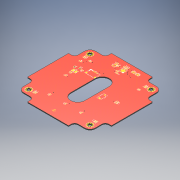
# Autodesk Inventor part: -ZPanel_PCB
Saved by Autodesk Inventor 2018 (Build 220112000, 112)
## iProperties
Created: 2018-11-03
Part Number: -ZPanel_PCB
Material: Epoxy Resin
Document SubType Name: Modeling
Designer: Bradley
Density: 1.14 g/cm^3
Appearance: Smooth - Dark Gray
Mass: 5.79181 g
Surface Area: 172.339 cm^2
Volume: 5.08053 cm^3
Author: Bradley
Autodesk Inventor part; units mm, degrees
ref_plane "YZ Plane" through (0, 0, 0) normal (1, 0, 0) x (0, 1, 0)
ref_plane "XZ Plane" through (0, 0, 0) normal (0, 1, 0) x (-1, 0, 0)
ref_plane "XY Plane" through (0, 0, 0) normal (0, 0, 1) x (1, 0, 0)
sketch "Sketch1" plane through (0, 0, 0) normal (0, 0, 1) x (1, 0, 0)
  line L0 (-48, -48) -> (48, -48)
  line L1 (48, -48) -> (48, 48)
  line L2 (48, 48) -> (-48, 48)
  line L3 (-48, 48) -> (-48, -48)
  line L4 (-48, -48) -> (48, 48) construction
  line L5 (48, -48) -> (-48, 48) construction
  circle A0 centre (0, 0) radius 40 construction
  circle A1 centre (0, 0) radius 8
  line L6 (-45, -32.5) -> (45, -32.5) construction
  line L7 (45, -32.5) -> (45, 32.5) construction
  line L8 (45, 32.5) -> (-45, 32.5) construction
  line L9 (-45, 32.5) -> (-45, -32.5) construction
  line L10 (-45, -32.5) -> (45, 32.5) construction
  line L11 (45, -32.5) -> (-45, 32.5) construction
  line L12 (-28, -46.5) -> (28, -46.5) construction
  line L13 (28, -46.5) -> (28, 46.5) construction
  line L14 (28, 46.5) -> (-28, 46.5) construction
  line L15 (-28, 46.5) -> (-28, -46.5) construction
  line L16 (-28, -46.5) -> (28, 46.5) construction
  line L17 (28, -46.5) -> (-28, 46.5) construction
  circle A2 centre (-45, 32.5) radius 4 construction
  circle A3 centre (-28, 46.5) radius 4 construction
  line L18 (-35, -35) -> (35, -35) construction
  line L19 (35, -35) -> (35, 35) construction
  line L20 (35, 35) -> (-35, 35) construction
  line L21 (-35, 35) -> (-35, -35) construction
  line L22 (-35, -35) -> (35, 35) construction
  line L23 (35, -35) -> (-35, 35) construction
  circle A4 centre (-35, 35) radius 3 construction
  line L24 (-23.5, 48) -> (-23.5, 45)
  arc A5 (-27.5, 41) -> (-23.5, 45) centre (-27.5, 45) ccw
  line L25 (-27.5, 41) -> (-35, 41)
  arc A6 (-35, 41) -> (-41, 35) centre (-35, 35) ccw
  line L26 (-41, 35) -> (-41, 27.5)
  arc A7 (-45, 23.5) -> (-41, 27.5) centre (-45, 27.5) ccw
  line L27 (-45, 23.5) -> (-48, 23.5)
  line L28 (48, 23.5) -> (45, 23.5)
  arc A8 (41, 27.5) -> (45, 23.5) centre (45, 27.5) ccw
  line L29 (41, 27.5) -> (41, 35)
  arc A9 (41, 35) -> (35, 41) centre (35, 35) ccw
  line L30 (35, 41) -> (27.5, 41)
  arc A10 (23.5, 45) -> (27.5, 41) centre (27.5, 45) ccw
  line L31 (23.5, 45) -> (23.5, 48)
  line L32 (48, -23.5) -> (45, -23.5)
  arc A11 (45, -23.5) -> (41, -27.5) centre (45, -27.5) ccw
  line L33 (41, -27.5) -> (41, -35)
  arc A12 (35, -41) -> (41, -35) centre (35, -35) ccw
  line L34 (35, -41) -> (27.5, -41)
  arc A13 (27.5, -41) -> (23.5, -45) centre (27.5, -45) ccw
  line L35 (23.5, -45) -> (23.5, -48)
  line L36 (-23.5, -48) -> (-23.5, -45)
  arc A14 (-23.5, -45) -> (-27.5, -41) centre (-27.5, -45) ccw
  line L37 (-27.5, -41) -> (-35, -41)
  arc A15 (-41, -35) -> (-35, -41) centre (-35, -35) ccw
  line L38 (-41, -35) -> (-41, -27.5)
  arc A16 (-41, -27.5) -> (-45, -23.5) centre (-45, -27.5) ccw
  line L39 (-45, -23.5) -> (-48, -23.5)
  line L40 (0, 14) -> (0, -14) construction
  line L41 (8, 14) -> (8, -14)
  line L42 (-8, -14) -> (-8, 14)
  arc A17 (8, 14) -> (-8, 14) centre (0, 14) ccw
  arc A18 (-8, -14) -> (8, -14) centre (0, -14) ccw
  dimension "d0" = 96
  dimension "d1" = 96
  dimension "d3" = 80
  dimension "d7" = 16
  dimension "d48" = 90
  dimension "d49" = 65
  dimension "d50" = 56
  dimension "d51" = 93
  dimension "d52" = 8
  dimension "d53" = 70
  dimension "d54" = 6
  dimension "d55" = 23.5
  dimension "d56" = 23.5
  dimension "d57" = 4
  dimension "d58" = 41
  dimension "d59" = 28
  constraints: 86 end point, 28 point on circle, 28 tangent, 19 centre point, 17 perpendicular, 11 equal radius, 11 point on line, 9 midpoint, 8 parallel, 7 collinear, 6 horizontal, 5 coincident, 4 equal length, 3 vertical, 1 concentric, 3 other
  measures "d0" distance of L2.end L1.end
  measures "d1" distance of L1.end L0.end
  measures "d3" diameter of A0
  measures "d7" diameter of A1
  measures "d48" distance of L8.end L7.end
  measures "d49" distance of L7.end L6.end
  measures "d50" distance of L14.end L14.start
  measures "d51" distance of L14.start L12.end
  measures "d52" diameter of A2
  measures "d53" distance of L20.end L19.end
  measures "d54" diameter of A4
  measures "d55" distance from line of point (0, 0) L24
  measures "d56" distance from line of point (0, 0) L27
  measures "d57" radius of A5
  measures "d58" distance from line of point (0, 0) L26
  measures "d59" distance of L41.start L41.end
extrude "Extrusion1" add sketch "Sketch1" along normal mid plane 1 contours L36 A14 L37 A15 L38 A16 L39 L3 L27 A7 L26 A6 L25 A5 L24 L2 L31 A10 L30 A9 L29 A8 L28 L1 L32 A11 L33 A12 L34 A13 L35 L0
fillet "Fillet1" radius 0.5 8 edges at (-23.5, -48, 0) (-48, -23.5, 0) (-48, 23.5, 0) (-23.5, 48, 0) (23.5, 48, 0) (48, 23.5, 0) (48, -23.5, 0) (23.5, -48, 0)
sketch "Sketch4" plane through (0, 0, 0.5) normal (0, 0, 1) x (1, 0, 0)
  line L0 (-35, -35) -> (35, -35) construction
  line L1 (35, -35) -> (35, 35) construction
  line L2 (35, 35) -> (-35, 35) construction
  line L3 (-35, 35) -> (-35, -35) construction
  line L4 (-35, -35) -> (35, 35) construction
  line L5 (35, -35) -> (-35, 35) construction
  point P0 (0, 0)
  dimension "d35" = 70
  constraints: 12 end point, 4 coincident, 2 midpoint, 2 parallel, 2 perpendicular, 1 horizontal
  measures "d35" distance of L2.end L1.end
hole "Hole3" at (-35, 35, 0.5) at (35, 35, 0.5) at (35, -35, 0.5) at (-35, -35, 0.5) direction (0, 0, -1) diameter 3.4 end through all clearance for "Flat Head Machine Screw" size "M3" standard "Ansi Metric M Profile"
sketch "Sketch13" plane through (0, 0, 0.5) normal (0, 0, 1) x (1, 0, 0)
  line L0 (-48, 48) -> (48, 48) construction
  line L1 (48, 48) -> (48, -48) construction
  line L2 (48, -48) -> (-48, -48) construction
  line L3 (-48, -48) -> (-48, 48) construction
  line L4 (23, 48) -> (-23, 48) projected
  line L5 (-23, -48) -> (23, -48) projected
  point P0 (0, 0)
  point P1 (0, 48)
  constraints: 2 collinear, 2 midpoint, 2 other
decal "Decal3"
sketch "Sketch8" plane through (0, 0, -0.5) normal (0, 0, -1) x (-1, 0, 0)
  line L0 (-48, 48) -> (48, 48) construction
  line L1 (48, 48) -> (48, -48) construction
  line L2 (48, -48) -> (-48, -48) construction
  line L3 (-48, -48) -> (-48, 48) construction
  line L4 (23, 48) -> (-23, 48) projected
  line L5 (-23, -48) -> (23, -48) projected
  point P0 (0, 0)
  point P1 (0, 48)
  constraints: 2 collinear, 2 midpoint, 2 other
decal "Decal2"
sketch "Sketch9" plane through (0, 0, 0.5) normal (0, 0, 1) x (1, 0, 0)
  point P0 (0, 0)
  point P1 (-26.75, 15.31)
  point P2 (-31.25, 13.5)
  constraints: 2 other
hole "Hole4" at (-26.75, 15.31, 0.5) at (-31.25, 13.5, 0.5) direction (0, 0, -1) diameter 0.7 end through all
sketch "Sketch10" plane through (0, 0, 0.5) normal (0, 0, 1) x (1, 0, 0)
  point P0 (0, 0)
  point P1 (35.711, -32.813)
  point P2 (34.289, -32.813)
  point P3 (33.139, -33.648)
  point P4 (32.7, -35)
  point P5 (34.289, -37.187)
  point P6 (35.711, -37.187)
  point P7 (36.861, -36.352)
  point P8 (37.3, 35)
  point P9 (-32.7, 35)
  point P10 (36.861, 36.352)
  point P11 (35.711, 37.187)
  point P12 (33.139, 36.352)
  point P13 (32.7, 35)
  point P14 (33.139, 33.648)
  point P15 (34.289, 32.813)
  point P16 (35.711, 32.813)
  point P17 (36.861, 33.648)
  point P18 (34.289, 37.187)
  point P19 (-32.7, -35)
  point P20 (-33.139, -33.648)
  point P21 (-34.289, -32.813)
  point P22 (-35.711, -32.813)
  point P23 (-36.861, -33.648)
  point P24 (-37.3, -35)
  point P25 (-36.861, -36.352)
  point P26 (-35.711, -37.187)
  point P27 (-34.289, -37.187)
  point P28 (-33.139, -36.352)
  point P29 (33.139, -36.352)
  point P30 (-33.139, 36.352)
  point P31 (-34.289, 37.187)
  point P32 (-35.711, 37.187)
  point P33 (-36.861, 36.352)
  point P34 (-37.3, 35)
  point P35 (-36.861, 33.648)
  point P36 (-35.711, 32.813)
  point P37 (-34.289, 32.813)
  point P38 (-33.139, 33.648)
  point P39 (37.3, -35)
  point P40 (36.861, -33.648)
  constraints: 41 other
hole "Hole5" at (35.711, -32.813, 0.5) at (34.289, -32.813, 0.5) at (33.139, -33.648, 0.5) at (32.7, -35, 0.5) at (34.289, -37.187, 0.5) at (35.711, -37.187, 0.5) at (36.861, -36.352, 0.5) at (37.3, 35, 0.5) at (-32.7, 35, 0.5) at (36.861, 36.352, 0.5) at (35.711, 37.187, 0.5) at (33.139, 36.352, 0.5) at (32.7, 35, 0.5) at (33.139, 33.648, 0.5) at (34.289, 32.813, 0.5) at (35.711, 32.813, 0.5) at (36.861, 33.648, 0.5) at (34.289, 37.187, 0.5) at (-32.7, -35, 0.5) at (-33.139, -33.648, 0.5) at (-34.289, -32.813, 0.5) at (-35.711, -32.813, 0.5) at (-36.861, -33.648, 0.5) at (-37.3, -35, 0.5) at (-36.861, -36.352, 0.5) at (-35.711, -37.187, 0.5) at (-34.289, -37.187, 0.5) at (-33.139, -36.352, 0.5) at (33.139, -36.352, 0.5) at (-33.139, 36.352, 0.5) at (-34.289, 37.187, 0.5) at (-35.711, 37.187, 0.5) at (-36.861, 36.352, 0.5) at (-37.3, 35, 0.5) at (-36.861, 33.648, 0.5) at (-35.711, 32.813, 0.5) at (-34.289, 32.813, 0.5) at (-33.139, 33.648, 0.5) at (37.3, -35, 0.5) at (36.861, -33.648, 0.5) direction (0, 0, -1) diameter 0.45 end through all
sketch "Sketch11" plane through (0, 0, 0.5) normal (0, 0, 1) x (1, 0, 0)
  point P0 (0, 0)
  point P1 (-11.75, 22.5)
  point P2 (-30.25, 22.5)
  point P3 (-4.025, 32.275)
  point P4 (-6.25, 34.75)
  point P5 (-29.5, 25.5)
  point P6 (-8, 23.5)
  point P7 (-6, 39.75)
  point P8 (5.25, 42.5)
  point P9 (2.5, 41.25)
  point P10 (-25, 28)
  point P11 (4.25, 39)
  point P12 (-25.75, 0)
  point P13 (4.75, 38)
  point P14 (-18, -23.5)
  point P15 (6, 37)
  point P16 (2, -25.25)
  point P17 (6.75, 36)
  point P18 (-11.75, 42.75)
  point P19 (25, 1.5)
  point P20 (11.5, 35)
  point P21 (18, -24.5)
  point P22 (9, 35.75)
  constraints: 23 other
hole "Hole6" at (-11.75, 22.5, 0.5) at (-30.25, 22.5, 0.5) at (-4.025, 32.275, 0.5) at (-6.25, 34.75, 0.5) at (-29.5, 25.5, 0.5) at (-8, 23.5, 0.5) at (-6, 39.75, 0.5) at (5.25, 42.5, 0.5) at (2.5, 41.25, 0.5) at (-25, 28, 0.5) at (4.25, 39, 0.5) at (-25.75, 0, 0.5) at (4.75, 38, 0.5) at (-18, -23.5, 0.5) at (6, 37, 0.5) at (2, -25.25, 0.5) at (6.75, 36, 0.5) at (-11.75, 42.75, 0.5) at (25, 1.5, 0.5) at (11.5, 35, 0.5) at (18, -24.5, 0.5) at (9, 35.75, 0.5) direction (0, 0, -1) diameter 0.35 end through all
equation "\"d56\" = d55"
body "Solid1"
